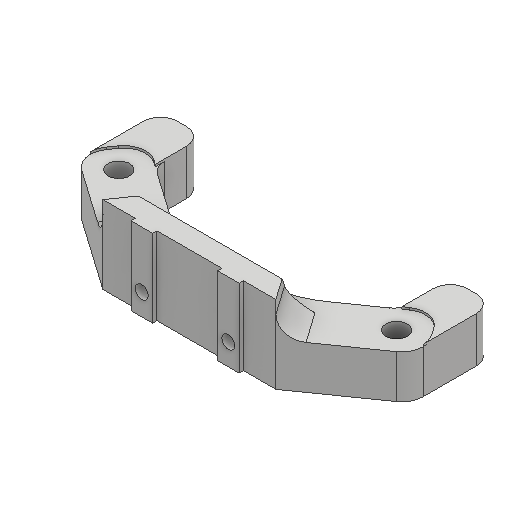
# Autodesk Inventor part: 3DP_PLA_Filament_Spool_Rollers
Saved by Autodesk Inventor 2026.1 (Build 301233000, 233)
## iProperties
Created: 2017-05-27
Part Number: 3DP_PLA_Filament_Spool_Rollers
Material: Ogólny
Document SubType Name: Modeling
Designer: Andrzej
Density: 1 g/cm^3
Appearance: Domyślna
Mass: 13.0166 g
Surface Area: 55.6585 cm^2
Volume: 13.0166 cm^3
Author: Andrzej
Autodesk Inventor part; units mm, degrees
ref_plane "YZ Plane" through (0, 0, 0) normal (1, 0, 0) x (0, 1, 0)
ref_plane "XZ Plane" through (0, 0, 0) normal (0, 1, 0) x (-1, 0, 0)
ref_plane "XY Plane" through (0, 0, 0) normal (0, 0, 1) x (1, 0, 0)
sketch "Szkic1" plane through (0, 0, 0) normal (0, 0, 1) x (1, 0, 0)
  line L0 (-4.1438, -2.0409) -> (35.8562, -2.0409)
  line L1 (35.8562, -2.0409) -> (56.335, 12.2985)
  line L2 (35.8562, -2.0409) -> (60.8562, -2.0409) construction
  line L3 (-4.1438, -2.0409) -> (-24.6226, 12.2985)
  line L4 (-4.1438, -2.0409) -> (20.8562, -2.0409) construction
  circle A0 centre (15.8562, 157.2218) radius 100
  line L5 (-24.6226, 12.2985) -> (-17.7397, 22.1283)
  line L6 (-17.7397, 22.1283) -> (2.7391, 7.7889)
  line L7 (56.335, 12.2985) -> (49.4521, 22.1283)
  line L8 (49.4521, 22.1283) -> (28.9733, 7.7889)
  line L9 (2.7391, 7.7889) -> (28.9733, 7.7889)
  point P0 (0, 0)
  point P1 (-16.2662, 13.7719)
  point P2 (47.9786, 13.7719)
  dimension "d0" = 40
  dimension "d1" = 25
  dimension "d2" = 35
  dimension "d3" = 25
  dimension "d4" = 145
  dimension "d5" = 200
  dimension "d6" = 20
  dimension "d7" = 12
  dimension "d8" = 25
  dimension "d9" = 12
  dimension "d10" = 25
  dimension "d11" = 6
  dimension "d12" = 6
  dimension "d13" = 6
  dimension "d14" = 6
  constraints: 20 end point, 4 horizontal, 2 equal length, 2 perpendicular, 1 centre point
  measures "d0" distance of L0.start L0.end
  measures "d1" distance of L0.end L1.end
  measures "d2" angle of L2 L1
  measures "d3" distance of L0.start L3.end
  measures "d4" angle of L4 L3
  measures "d5" diameter of A0
  measures "d6" horizontal distance of L0.end A0.centre
  measures "d7" distance of L3.end L5.end
  measures "d8" distance of L5.end L6.end
  measures "d9" distance of L1.end L7.end
  measures "d10" distance of L7.end L8.end
  measures "d11" distance from line of L6 point (-16.266, 13.772)
  measures "d12" distance from line of L8 point (47.979, 13.772)
  measures "d13" distance from line of L5 point (-16.266, 13.772)
  measures "d14" distance from line of L7 point (47.979, 13.772)
extrude "Wyciągnięcie proste1" add sketch "Szkic1" along normal blind 10 contours L3 L5 L6 L9 L8 L7 L1 L0
hole "Otwór1" at (-16.2662, 13.7719, 0) at (47.9786, 13.7719, 0) direction (0, 0, 1) diameter 5 end through all
sketch "Szkic2" plane through (0, 0, 10) normal (0, 0, 1) x (1, 0, 0)
  circle A0 centre (-16.2662, 13.7719) radius 2.5 projected
  circle A1 centre (47.9786, 13.7719) radius 2.5 projected
  line L0 (-4.1438, -2.0409) -> (35.8562, -2.0409) projected
  line L1 (35.8562, -2.0409) -> (56.335, 12.2985) projected
  line L2 (56.335, 12.2985) -> (49.4521, 22.1283) projected
  line L3 (49.4521, 22.1283) -> (28.9733, 7.7889) projected
  line L4 (28.9733, 7.7889) -> (2.7391, 7.7889) projected
  line L5 (2.7391, 7.7889) -> (-17.7397, 22.1283) projected
  line L6 (-17.7397, 22.1283) -> (-24.6226, 12.2985) projected
  line L7 (-24.6226, 12.2985) -> (-4.1438, -2.0409) projected
  line L8 (2.7391, 7.7889) -> (-17.7397, 22.1283) projected
  line L9 (2.7391, 7.7889) -> (-4.1438, -2.0409)
  line L10 (28.9733, 7.7889) -> (35.8562, -2.0409)
  point P0 (0, 0)
  constraints: 4 end point, 2 perpendicular
extrude "Wyciągnięcie proste2" add sketch "Szkic2" along normal blind 8 contours L9 L4 L10 L0
chamfer "Faza1" distance 5 distance2 8 1 edges at (15.8562, 7.7889, 18) measured on face at (20.2286, 1.2357, 18)
fillet "Zaokrąglenie1" radius 20 2 edges at (2.7391, 7.7889, 5) (28.9733, 7.7889, 5)
fillet "Zaokrąglenie1" radius 5 4 edges at (-17.7397, 22.1283, 5) (-24.6226, 12.2985, 5) (49.4521, 22.1283, 5) (56.335, 12.2985, 5)
fillet "Zaokrąglenie2" radius 5 2 edges at (-0.7023, 2.874, 10) (32.4148, 2.874, 10)
sketch "Szkic3" plane through (9.0451, 7.7889, 0) normal (0, 1, 0) x (1, 0, 0)
  line L0 (13.6222, 0) -> (13.6222, -10) projected
  line L1 (13.6222, 0) -> (0, 0) projected
  line L2 (0, -10) -> (0, 0) projected
  line L3 (13.6222, -10) -> (0, -10) projected
  circle A0 centre (-3.1889, -5) radius 1.5
  circle A1 centre (16.8111, -5) radius 1.5
  circle A2 centre (-3.1889, -5) radius 3.5
  circle A3 centre (16.8111, -5) radius 3.5
  point P0 (-9.0451, 0)
  dimension "d32" = 20
  dimension "d33" = 10
  dimension "d34" = 5
  dimension "d35" = 5
  dimension "d36" = 13.6222
  dimension "d37" = 3.1889
  dimension "d38" = 3
  dimension "d39" = 3
  dimension "d40" = 7
  dimension "d41" = 7
  constraints: 4 centre point, 4 coincident
  measures "d32" distance of point (16.811, -5) point (-3.189, -5)
  measures "d33" distance between parallel lines of L1 L3
  measures "d34" distance from line of L1 point (-3.189, -5)
  measures "d35" distance from line of L1 point (16.811, -5)
  measures "d36" distance between parallel lines of L0 L2
  measures "d37" distance from line of L2 point (-3.189, -5)
  measures "d38" diameter of A0
  measures "d39" diameter of A1
  measures "d40" diameter of A2
  measures "d41" diameter of A3
extrude "Wyciągnięcie proste3" cut sketch "Szkic3" along normal mid plane 20 contours A0 | A1
extrude "Wyciągnięcie proste4" cut sketch "Szkic3" along normal blind 20 contours A3 L0 | L0 A3 | A2 L2 | L2 A2
sketch "Szkic4" plane through (0, 0, 0) normal (0, 0, -1) x (-1, 0, 0)
  arc A0 (-53.4671, 16.3942) -> (-52.2393, 9.4306) centre (-49.3714, 13.5263) ccw projected
  line L0 (-35.8562, -2.0409) -> (-52.2393, 9.4306) projected
  line L1 (4.1438, -2.0409) -> (-35.8562, -2.0409) projected
  line L2 (20.5268, 9.4306) -> (4.1438, -2.0409) projected
  arc A1 (20.5268, 9.4306) -> (21.7547, 16.3942) centre (17.6589, 13.5263) ccw projected
  line L3 (20.6076, 18.0325) -> (21.7547, 16.3942) projected
  arc A2 (20.6076, 18.0325) -> (13.6439, 19.2604) centre (16.5118, 15.1646) ccw projected
  line L4 (2.4264, 11.4058) -> (13.6439, 19.2604) projected
  arc A3 (-9.0451, 7.7889) -> (2.4264, 11.4058) centre (-9.0451, 27.7889) ccw projected
  line L5 (-22.6673, 7.7889) -> (-9.0451, 7.7889) projected
  arc A4 (-34.1388, 11.4058) -> (-22.6673, 7.7889) centre (-22.6673, 27.7889) ccw projected
  line L6 (-45.3563, 19.2604) -> (-34.1388, 11.4058) projected
  arc A5 (-45.3563, 19.2604) -> (-52.32, 18.0325) centre (-48.2242, 15.1646) ccw projected
  line L7 (-53.4671, 16.3942) -> (-52.32, 18.0325) projected
  circle A6 centre (-47.9786, 13.7719) radius 2.5 projected
  circle A7 centre (16.2662, 13.7719) radius 2.5 projected
  line L8 (-54.3714, 13.5263) -> (-54.3714, 29.7719)
  line L9 (-54.3714, 29.7719) -> (-44.3714, 29.7719)
  line L10 (-44.3714, 29.7719) -> (-44.3714, 18.5707)
  line L11 (12.6589, 18.5707) -> (12.6589, 29.7719)
  line L12 (12.6589, 29.7719) -> (22.6589, 29.7719)
  line L13 (22.6589, 29.7719) -> (22.6589, 13.5263)
  arc A8 (20.5268, 9.4306) -> (21.7547, 16.3942) centre (17.6589, 13.5263) ccw projected
  point P0 (0, 0)
  dimension "d46" = 16
  dimension "d47" = 16
  dimension "d48" = 10
  dimension "d49" = 10
  constraints: 12 end point, 3 perpendicular, 3 vertical, 2 point on circle, 2 point on line, 2 tangent
  measures "d46" distance from line of A6.centre L9
  measures "d47" distance from line of A7.centre L12
  measures "d48" distance between parallel lines of L10 L8
  measures "d49" distance of L11.end L12.end
extrude "Wyciągnięcie proste5" add sketch "Szkic4" against normal blind 10.5 contours A0 L8 L9 L10 L6 A5 L7 | A1 L3 A2 L4 L11 L12 L13
fillet "Zaokrąglenie3" radius 4 4 edges at (54.3714, 29.7719, 5.25) (44.3714, 29.7719, 5.25) (-12.6589, 29.7719, 5.25) (-22.6589, 29.7719, 5.25)
fillet "Zaokrąglenie4" radius 4 2 edges at (-12.6589, 18.5707, 5) (44.3714, 18.5707, 5)
sketch "Szkic5" plane through (-4.1438, -2.0409, 0) normal (0, -1, 0) x (1, 0, 0)
  circle A0 centre (10, 5) radius 1.5 projected
  circle A1 centre (30, 5) radius 1.5 projected
  line L0 (0, 0) -> (40, 0) projected
  line L1 (40, 0) -> (40, 15) projected
  line L2 (40, 15) -> (40, 18) projected
  line L3 (0, 18) -> (40, 18) projected
  line L4 (0, 15) -> (0, 18) projected
  line L5 (0, 0) -> (0, 15) projected
  line L6 (7.5, 18) -> (7.5, 0)
  line L7 (3.3819, 18) -> (36.6181, 18) projected
  line L8 (12.5, 18) -> (12.5, 0)
  line L9 (0, 0) -> (40, 0) projected
  line L10 (27.5, 18) -> (27.5, 0)
  line L11 (32.5, 18) -> (32.5, 0)
  point P0 (4.1438, 0)
  dimension "d54" = 40
  dimension "d55" = 5
  dimension "d56" = 5
  dimension "d57" = 7.5
  dimension "d58" = 7.5
  constraints: 8 end point, 8 point on line, 3 perpendicular, 1 parallel
  measures "d54" distance between parallel lines of L1 L4
  measures "d55" distance between parallel lines of L8 L6
  measures "d56" distance between parallel lines of L11 L10
  measures "d57" distance between parallel lines of L5 L6
  measures "d58" distance between parallel lines of L1 L11
extrude "Wyciągnięcie proste6" add sketch "Szkic5" along normal blind 1 contours L6 L3 L8 L0 | L10 L3 L11 L0
equation "\"d1\" = d3"
equation "\"d8\" = d3"
equation "\"d9\" = d7"
equation "\"d10\" = d3"
equation "\"d11\" = 0.5 * d7"
equation "\"d12\" = d11"
equation "\"d34\" = 0.5 * d33"
equation "\"d35\" = d34"
equation "\"d37\" = -0.5 * d36 + 0.5 * d32"
equation "\"d47\" = d46"
equation "\"d49\" = d48"
equation "\"d58\" = d57"
